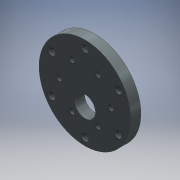
# Autodesk Inventor part: motor_mounting_plate
Saved by Autodesk Inventor 2016 (Build 200138000, 138)
## iProperties
Created: 2016-12-26
Part Number: motor_mounting_plate
Material: Generic
Document SubType Name: Modeling
Designer: hesaon
Density: 1 g/cm^3
Appearance: Default
Author: hesaon
Autodesk Inventor part; units mm, degrees
ref_plane "YZ Plane" through (0, 0, 0) normal (1, 0, 0) x (0, 1, 0)
ref_plane "XZ Plane" through (0, 0, 0) normal (0, 1, 0) x (-1, 0, 0)
ref_plane "XY Plane" through (0, 0, 0) normal (0, 0, 1) x (1, 0, 0)
sketch "Sketch1" plane through (0, 0, 0) normal (0, 1, 0) x (-1, 0, 0)
  circle A0 centre (0, 0) radius 27.5
  circle A1 centre (0, -7) radius 6.25
  circle A2 centre (15.5, 0) radius 1.6
  circle A3 centre (7.75, 13.4234) radius 1.6
  circle A4 centre (-7.75, 13.4234) radius 1.6
  circle A5 centre (-15.5, 0) radius 1.6
  circle A6 centre (-7.75, -13.4234) radius 1.6
  circle A7 centre (7.75, -13.4234) radius 1.6
  circle A8 centre (0, 23) radius 2.1
  circle A9 centre (-19.9186, 11.5) radius 2.1
  circle A10 centre (-19.9186, -11.5) radius 2.1
  circle A11 centre (0, -23) radius 2.1
  circle A12 centre (19.9186, -11.5) radius 2.1
  circle A13 centre (19.9186, 11.5) radius 2.1
  dimension "d0" = 55
  dimension "d1" = 12.5
  dimension "d2" = 7
  dimension "d3" = 3.2
  dimension "d4" = 15.5
  dimension "d7" = 360
  dimension "d9" = 4.2
  dimension "d10" = 23
  dimension "d13" = 360
  constraints: 14 centre point, 2 vertical alignment, 1 coincident, 1 horizontal alignment, 26 other
  measures "d0" diameter of A0
  measures "d1" diameter of A1
  measures "d2" distance of point (0, 0) A1.centre
  measures "d3" diameter of A2
  measures "d4" distance of A2.centre point (0, 0)
  measures "d9" diameter of A8
  measures "d10" distance of point (0, 0) A8.centre
extrude "Extrusion1" add sketch "Sketch1" along normal blind 6
body "Solid1"
